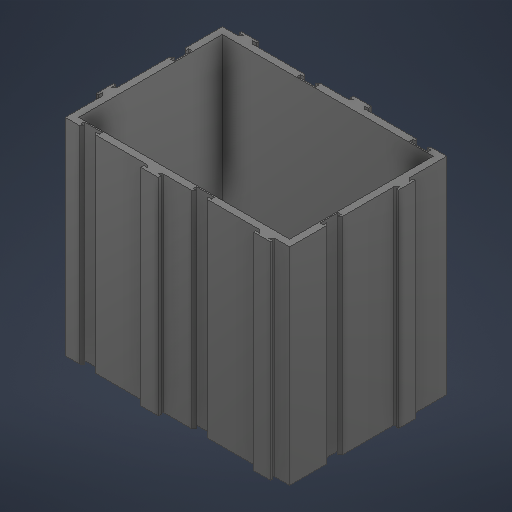
# Autodesk Inventor part: box1x2
Saved by Autodesk Inventor 2027 (Build 310192060, 192F)
## iProperties
Created: 2026-06-08
Part Number: box1x2
Material: Ogólny
Document SubType Name: Modeling
Designer: User
Density: 1 g/cm^3
Appearance: Domyślna
Author: User
Autodesk Inventor part; units mm, degrees
ref_plane "YZ Plane" through (0, 0, 0) normal (1, 0, 0) x (0, 1, 0)
ref_plane "XZ Plane" through (0, 0, 0) normal (0, 1, 0) x (-1, 0, 0)
ref_plane "XY Plane" through (0, 0, 0) normal (0, 0, 1) x (1, 0, 0)
sketch "Szkic1" plane through (0, 0, 0) normal (0, 1, 0) x (-1, 0, 0)
  line L0 (-50, -35) -> (50, -35)
  line L1 (50, -35) -> (50, 35)
  line L2 (50, 35) -> (-50, 35)
  line L3 (-50, 35) -> (-50, -35)
  line L4 (-50, -35) -> (50, 35) construction
  line L5 (50, -35) -> (-50, 35) construction
  line L6 (-47, -32) -> (47, -32)
  line L7 (47, -32) -> (47, 32)
  line L8 (47, 32) -> (-47, 32)
  line L9 (-47, 32) -> (-47, -32)
  line L10 (-47, -32) -> (47, 32) construction
  line L11 (47, -32) -> (-47, 32) construction
  line L12 (50, 35) -> (43.5607, 35)
  line L13 (50, 35) -> (56.4393, 35) construction
  line L14 (43.5607, 35) -> (42.5, 33.9393)
  line L15 (42.5, 33.9393) -> (44, 33.9393)
  line L16 (44, 33.9393) -> (44, 32.5393)
  line L17 (-50, 35) -> (-48, 35) construction
  line L18 (0, 32) -> (0, 35) construction
  line L19 (43.5607, 35) -> (60.1482, 35) construction
  line L20 (36.4393, 35) -> (57.1482, 35) construction
  line L21 (44, 32.5393) -> (40, 32.5393)
  line L22 (40, 32.5393) -> (40, 35) construction
  line L23 (36.4393, 35) -> (37.5, 33.9393)
  line L24 (37.5, 33.9393) -> (36, 33.9393)
  line L25 (36, 33.9393) -> (36, 32.5393)
  line L26 (36, 32.5393) -> (40, 32.5393)
  line L27 (-43.5607, 35) -> (-42.5, 33.9393) construction
  line L28 (-42.5, 33.9393) -> (-44, 33.9393) construction
  line L29 (-44, 32.5393) -> (-40, 32.5393) construction
  line L30 (-40, 32.5393) -> (-40, 35) construction
  line L31 (-36.4393, 35) -> (-37.5, 33.9393) construction
  line L32 (-36, 32.5393) -> (-40, 32.5393) construction
  line L33 (-36, 33.9393) -> (-36, 32.5393) construction
  line L34 (-37.5, 33.9393) -> (-36, 33.9393) construction
  line L35 (-44, 33.9393) -> (-44, 32.5393) construction
  line L36 (47, 0) -> (-47, 0) construction
  line L37 (50, 0) -> (47, 0) construction
  line L38 (43.5607, -35) -> (42.5, -33.9393) construction
  line L39 (42.5, -33.9393) -> (44, -33.9393) construction
  line L40 (44, -33.9393) -> (44, -32.5393) construction
  line L41 (44, -32.5393) -> (40, -32.5393) construction
  line L42 (40, -32.5393) -> (40, -35) construction
  line L43 (36.4393, -35) -> (37.5, -33.9393) construction
  line L44 (36, -32.5393) -> (40, -32.5393) construction
  line L45 (36, -33.9393) -> (36, -32.5393) construction
  line L46 (37.5, -33.9393) -> (36, -33.9393) construction
  line L47 (-36.4393, -35) -> (-37.5, -33.9393)
  line L48 (-37.5, -33.9393) -> (-36, -33.9393)
  line L49 (-40, -32.5393) -> (-40, -35) construction
  line L50 (-36, -32.5393) -> (-40, -32.5393)
  line L51 (-43.5607, -35) -> (-42.5, -33.9393)
  line L52 (-42.5, -33.9393) -> (-44, -33.9393)
  line L53 (-44, -32.5393) -> (-40, -32.5393)
  line L54 (-36, -33.9393) -> (-36, -32.5393)
  line L55 (-44, -33.9393) -> (-44, -32.5393)
  line L56 (50, 11.4393) -> (48.9393, 12.5) construction
  line L57 (48.9393, 12.5) -> (48.9393, 11) construction
  line L58 (48.9393, 11) -> (47.5393, 11) construction
  line L59 (47.5393, 11) -> (47.5393, 15) construction
  line L60 (47.5393, 15) -> (49.8, 15) construction
  line L61 (50, 18.5607) -> (48.9393, 17.5) construction
  line L62 (47.5393, 19) -> (47.5393, 15) construction
  line L63 (48.9393, 19) -> (47.5393, 19) construction
  line L64 (48.9393, 17.5) -> (48.9393, 19) construction
  line L65 (50, -11.4393) -> (48.9393, -12.5)
  line L66 (48.9393, -12.5) -> (48.9393, -11)
  line L67 (48.9393, -11) -> (47.5393, -11)
  line L68 (47.5393, -11) -> (47.5393, -15)
  line L69 (50, -18.5607) -> (48.9393, -17.5)
  line L70 (48.9393, -17.5) -> (48.9393, -19)
  line L71 (47.5393, -15) -> (49.8, -15) construction
  line L72 (47.5393, -19) -> (47.5393, -15)
  line L73 (48.9393, -19) -> (47.5393, -19)
  line L74 (-50, 11.4393) -> (-48.9393, 12.5)
  line L75 (-48.9393, 12.5) -> (-48.9393, 11)
  line L76 (-48.9393, 11) -> (-47.5393, 11)
  line L77 (-47.5393, 11) -> (-47.5393, 15)
  line L78 (-50, 18.5607) -> (-48.9393, 17.5)
  line L79 (-48.9393, 17.5) -> (-48.9393, 19)
  line L80 (-47.5393, 15) -> (-49.8, 15) construction
  line L81 (-47.5393, 19) -> (-47.5393, 15)
  line L82 (-48.9393, 19) -> (-47.5393, 19)
  line L83 (-50, -11.4393) -> (-48.9393, -12.5) construction
  line L84 (-48.9393, -12.5) -> (-48.9393, -11) construction
  line L85 (-48.9393, -11) -> (-47.5393, -11) construction
  line L86 (-47.5393, -11) -> (-47.5393, -15) construction
  line L87 (-47.5393, -15) -> (-49.8, -15) construction
  line L88 (-50, -18.5607) -> (-48.9393, -17.5) construction
  line L89 (-47.5393, -19) -> (-47.5393, -15) construction
  line L90 (-48.9393, -17.5) -> (-48.9393, -19) construction
  line L91 (-48.9393, -19) -> (-47.5393, -19) construction
  line L92 (-36.4393, 35) -> (-37.5, 36.0607)
  line L93 (-37.5, 36.0607) -> (-36, 36.0607)
  line L94 (-40, 37.4607) -> (-40, 35)
  line L95 (-36, 37.4607) -> (-40, 37.4607)
  line L96 (-43.5607, 35) -> (-42.5, 36.0607)
  line L97 (-42.5, 36.0607) -> (-44, 36.0607)
  line L98 (-44, 37.4607) -> (-40, 37.4607)
  line L99 (-36, 36.0607) -> (-36, 37.4607)
  line L100 (-44, 36.0607) -> (-44, 37.4607)
  line L101 (43.5607, -35) -> (42.5, -36.0607)
  line L102 (42.5, -36.0607) -> (44, -36.0607)
  line L103 (44, -36.0607) -> (44, -37.4607)
  line L104 (44, -37.4607) -> (40, -37.4607)
  line L105 (36, -37.4607) -> (40, -37.4607)
  line L106 (40, -37.4607) -> (40, -35) construction
  line L107 (36.4393, -35) -> (37.5, -36.0607)
  line L108 (36, -36.0607) -> (36, -37.4607)
  line L109 (37.5, -36.0607) -> (36, -36.0607)
  line L110 (50, 11.4393) -> (51.0607, 12.5)
  line L111 (51.0607, 12.5) -> (51.0607, 11)
  line L112 (51.0607, 11) -> (52.4607, 11)
  line L113 (52.4607, 11) -> (52.4607, 15)
  line L114 (50, 18.5607) -> (51.0607, 17.5)
  line L115 (51.0607, 17.5) -> (51.0607, 19)
  line L116 (52.4607, 15) -> (50.2, 15) construction
  line L117 (52.4607, 19) -> (52.4607, 15)
  line L118 (51.0607, 19) -> (52.4607, 19)
  line L119 (-51.0607, -19) -> (-52.4607, -19)
  line L120 (-51.0607, -17.5) -> (-51.0607, -19)
  line L121 (-50, -18.5607) -> (-51.0607, -17.5)
  line L122 (-52.4607, -11) -> (-52.4607, -15)
  line L123 (-52.4607, -15) -> (-50.2, -15) construction
  line L124 (-51.0607, -11) -> (-52.4607, -11)
  line L125 (-51.0607, -12.5) -> (-51.0607, -11)
  line L126 (-50, -11.4393) -> (-51.0607, -12.5)
  line L127 (-52.4607, -19) -> (-52.4607, -15)
  line L128 (-14, 33.9393) -> (-14, 32.5393)
  line L129 (-12.5, 33.9393) -> (-14, 33.9393)
  line L130 (-13.5607, 35) -> (-12.5, 33.9393)
  line L131 (-14, 32.5393) -> (-10, 32.5393)
  line L132 (-10, 32.5393) -> (-10, 35) construction
  line L133 (-6, 32.5393) -> (-10, 32.5393)
  line L134 (-6, 33.9393) -> (-6, 32.5393)
  line L135 (-7.5, 33.9393) -> (-6, 33.9393)
  line L136 (-6.4393, 35) -> (-7.5, 33.9393)
  line L137 (10, 37.4607) -> (10, 35)
  line L138 (14, 37.4607) -> (10, 37.4607)
  line L139 (14, 36.0607) -> (14, 37.4607)
  line L140 (13.5607, 35) -> (12.5, 36.0607)
  line L141 (12.5, 36.0607) -> (14, 36.0607)
  line L142 (6, 37.4607) -> (10, 37.4607)
  line L143 (6.4393, 35) -> (7.5, 36.0607)
  line L144 (6, 36.0607) -> (6, 37.4607)
  line L145 (7.5, 36.0607) -> (6, 36.0607)
  line L146 (0, -32) -> (0, -35) construction
  line L147 (14, -33.9393) -> (14, -32.5393)
  line L148 (13.5607, -35) -> (12.5, -33.9393)
  line L149 (12.5, -33.9393) -> (14, -33.9393)
  line L150 (10, -32.5393) -> (10, -35) construction
  line L151 (6.4393, -35) -> (7.5, -33.9393)
  line L152 (7.5, -33.9393) -> (6, -33.9393)
  line L153 (6, -33.9393) -> (6, -32.5393)
  line L154 (-14, -36.0607) -> (-14, -37.4607)
  line L155 (-13.5607, -35) -> (-12.5, -36.0607)
  line L156 (-12.5, -36.0607) -> (-14, -36.0607)
  line L157 (-14, -37.4607) -> (-10, -37.4607)
  line L158 (-6.4393, -35) -> (-7.5, -36.0607)
  line L159 (-7.5, -36.0607) -> (-6, -36.0607)
  line L160 (-6, -37.4607) -> (-10, -37.4607)
  line L161 (-6, -36.0607) -> (-6, -37.4607)
  line L162 (-10, -37.4607) -> (-10, -35)
  line L163 (6, -32.5393) -> (14, -32.5393)
  point P0 (0, 0)
  point P1 (-36.4393, 35)
  point P2 (-43.5607, 35)
  point P3 (-43.5607, -35)
  point P4 (-36.4393, -35)
  point P5 (36.4393, -35)
  point P6 (43.5607, -35)
  point P7 (43.5607, 35)
  point P8 (0, 33.5)
  point P9 (40, 33.7697)
  point P10 (48.5, 0)
  point P11 (-40, 33.7697)
  point P12 (48.6697, 15)
  point P13 (48.6697, -15)
  point P14 (-48.6697, 15)
  point P15 (-48.6697, -15)
  point P16 (48.6697, -15)
  point P17 (-50, 18.5607)
  point P18 (-50, 11.4393)
  point P19 (-50, -11.4393)
  point P20 (-50, -18.5607)
  point P21 (50, -18.5607)
  point P22 (50, -11.4393)
  point P23 (-40, 36.2303)
  point P24 (51.3303, 15)
  point P25 (-51.3303, -15)
  point P26 (-50, -18.5607)
  point P27 (-50, -11.4393)
  point P28 (43.5607, -35)
  point P29 (36.4393, -35)
  point P30 (-43.5607, 35)
  point P31 (-36.4393, 35)
  point P32 (-10, 33.7697)
  point P33 (-6.4393, 35)
  point P34 (-13.5607, 35)
  point P35 (10, 36.2303)
  point P36 (6.4393, 35)
  point P37 (13.5607, 35)
  point P38 (0, -33.5)
  point P39 (10, -33.7697)
  point P40 (-10, -36.2303)
  point P41 (-13.5607, -35)
  point P42 (-6.4393, -35)
  point P43 (6.4393, -35)
  point P44 (13.5607, -35)
  dimension "d0" = 100
  dimension "d1" = 70
  dimension "d2" = 94
  dimension "d3" = 64
  dimension "d6" = 1.5
  dimension "d7" = 135
  dimension "d8" = 1.5
  dimension "d9" = 1.4
  dimension "d15" = 2
  dimension "d23" = 4
  dimension "d29" = 45
  dimension "d34" = 1.5
  dimension "d35" = 1.5
  dimension "d36" = 1.4
  dimension "d37" = 4
  dimension "d38" = 45
  dimension "d76" = 1.1303
  dimension "d90" = 10
  dimension "d91" = 20
  dimension "d94" = 50
  dimension "d101" = 50
  dimension "d108" = 360
  constraints: 328 end point, 102 symmetric about line, 15 midpoint, 11 parallel, 7 point on line, 6 horizontal, 4 perpendicular, 2 collinear, 2 vertical, 125 other
  measures "d0" distance of L2.end L1.end
  measures "d1" distance of L1.end L0.end
  measures "d2" distance of L8.end L7.end
  measures "d3" distance of L7.end L6.end
  measures "d6" distance of L12.end L14.end
  measures "d7" angle of L14 L12
  measures "d8" distance of L14.end L15.end
  measures "d9" distance of L15.end L16.end
  measures "d15" distance of L2.end L17.end
  measures "d23" distance of L16.end L21.end
  measures "d29" angle of L24 L23
  measures "d34" distance of L56.start L56.end
  measures "d35" distance of L56.end L57.end
  measures "d36" distance of L57.end L58.end
  measures "d37" distance of L58.end L59.end
  measures "d38" angle of L64 L61
  measures "d76" distance of L68.end point (48.67, -15)
  measures "d90" distance from line of L1 point (40, 33.77)
  measures "d91" distance from line of L2 point (48.67, 15)
  measures "d94" distance of L26.start L128.end
  measures "d101" distance of L95.end L137.start
extrude "Wyciągnięcie proste1" add sketch "Szkic1" along normal blind 90 contours L3 L74 L75 L76 L77 L81 L82 L79 L78 L2 L130 L129 L128 L131 L133 L134 L135 L136 L23 L24 L25 L26 L21 L16 L15 L14 L1 L65 L66 L67 L68 L72 L73 L70 L69 L0 L148 L149 L147 L163 L153 L152 L151 L47 L48 L54 L50 L53 L55 L52 L51 | L121 L120 L119 L127 L122 L124 L125 L126 L3 | L0 L162 L157 L154 L156 L155 | L0 L158 L159 L161 L160 L162 | L96 L97 L100 L98 L94 L2 | L94 L95 L99 L93 L92 L2 | L0 L101 L102 L103 L104 L105 L108 L109 L107 | L143 L145 L144 L142 L137 L2 | L137 L138 L139 L141 L140 L2 | L1 L114 L115 L118 L117 L113 L112 L111 L110
extrude "Wyciągnięcie proste2" add sketch "Szkic1" against normal blind 2 contours L3 L74 L75 L76 L77 L81 L82 L79 L78 L2 L130 L129 L128 L131 L133 L134 L135 L136 L23 L24 L25 L26 L21 L16 L15 L14 L1 L65 L66 L67 L68 L72 L73 L70 L69 L0 L148 L149 L147 L163 L153 L152 L151 L47 L48 L54 L50 L53 L55 L52 L51 | L121 L120 L119 L127 L122 L124 L125 L126 L3 | L0 L162 L157 L154 L156 L155 | L0 L158 L159 L161 L160 L162 | L96 L97 L100 L98 L94 L2 | L94 L95 L99 L93 L92 L2 | L0 L101 L102 L103 L104 L105 L108 L109 L107 | L143 L145 L144 L142 L137 L2 | L137 L138 L139 L141 L140 L2 | L1 L114 L115 L118 L117 L113 L112 L111 L110 | L9 L8 L7 L6
offset faces "Rozmiar1" outward -0.2 faces at (-44, 59.3333, -36.5273) (-43.2071, 59.3333, -35.3536) (-41.3333, 59.3333, -37.4607) (-36, 59.3333, -36.994) (-37.1464, 59.3333, -35.7071) (-36.5, 59.3333, -36.0607) (-43, 59.3333, -36.0607) (-51.0607, 59.3333, 11.5) (-51.5273, 59.3333, 11) (-50.7071, 59.3333, 17.8536) (-51.994, 59.3333, 19) (-51.0607, 59.3333, 18) (-50.7071, 59.3333, 12.1464) (-52.4607, 28.6667, 13.6667) (38.6667, 28.6667, 37.4607) (44, 59.3333, 36.5273) (43.2071, 59.3333, 35.3536) (43, 59.3333, 36.0607) (36.5, 59.3333, 36.0607) (36, 59.3333, 36.994) (37.1464, 59.3333, 35.7071) (51.0607, 28.6667, -12) (51.5273, 59.3333, -11) (52.4607, 59.3333, -16.3333) (51.994, 59.3333, -19) (51.0607, 59.3333, -18)
move faces "Przesuń1" translate (0.05, 0, 0) faces at (51.2607, 28.6667, -18.3) (51.2607, 28.6667, -12.2) (52.2607, 28.6667, -13.7333)
move faces "Przesuń2" translate (-0.05, 0, 0) faces at (-51.2607, 28.6667, 18.2057) (-51.2607, 28.6667, 12.3886) (-52.2607, 28.6667, 13.7333)
move faces "Przesuń3" translate (0, 0, -0.05) faces at (-36.7943, 59.3333, -36.2607) (-42.6114, 59.3333, -36.2607) (-38.7333, 28.6667, -37.2607)
move faces "Przesuń4" translate (0, 0, 0.05) faces at (38.7333, 28.6667, 37.2607) (42.6114, 59.3333, 36.2607) (36.7943, 59.3333, 36.2607)
equation "\"Offcenter\" = 15"
